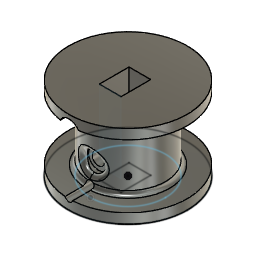
spool (Autodesk Fusion 360 design; units mm, degrees)
Autodesk Fusion 360 part; units mm, degrees
sketch "Skizze1" plane through (0, 0, 0) normal (0, 0, 1) x (1, 0, 0)
  circle A0 centre (0, 0) radius 15
  line L0 (-2.75, 3) -> (2.75, 3)
  line L1 (2.75, 3) -> (2.75, -4.5)
  line L2 (2.75, -4.5) -> (-2.75, -4.5)
  line L3 (-2.75, -4.5) -> (-2.75, 3)
  circle A1 centre (0, 0) radius 9.5
  point P0 (0, -9.5)
  dimension "d1" = 30
  dimension "d2" = 7.5
  dimension "d3" = 5.5
  dimension "d4" = 3
  dimension "d5" = 2.75
  dimension "d6" = 2.75
  dimension "d7" = 4.5
  dimension "d15" = 5
  constraint coincident A0.centre A1.centre
  constraint horizontal L0
  constraint vertical L1
  constraint horizontal L2
  constraint vertical L3
  constraint coincident A1 P0
  measures "d1" diameter of A0
  measures "d2" distance of L0 L2
  measures "d3" distance of L0.start L0.end
  measures "d4" distance of L0 A0.centre
  measures "d5" distance of L1 A0.centre
  measures "d6" distance of A0.centre L3
  measures "d7" distance of A0.centre L2
  measures "d15" distance of L2 P0
extrude "Extrusion1" add sketch "Skizze1" along normal blind 21 contours A0 | A1
extrude "Extrusion2" add sketch "Skizze1" along normal blind 3 contours L0 L1 L2 L3
hole "Bohrung1" at (0, 0, 0) direction (0, 0, 1) diameter 3.5 depth 6 tip angle 180
extrude "Extrusion3" cut sketch "Skizze1" along normal blind 16 from surface at 2.5 contours A0
sketch "Skizze2" plane through (0, -4.5, 0) normal (0, 1, 0) x (-1, 0, 0)
  line L0 (-2.75, 3) -> (2.75, 3)
  line L1 (2.75, 3) -> (2.75, 21)
  line L2 (2.75, 21) -> (-2.75, 21)
  line L3 (-2.75, 21) -> (-2.75, 3)
hole "Bohrung2" at (0, -9.5, 17.5) direction (0, 1, 0) diameter 3.1 depth 6 tip angle 180 counterbore diameter 5 counterbore depth 2
hole "Bohrung3" at (0, -9.5, 7.5) direction (0, 1, 0) diameter 3.1 depth 6 tip angle 180 counterbore diameter 5 counterbore depth 2
sketch "Skizze3" plane through (0, -4.5, 0) normal (0, 1, 0) x (-1, 0, 0)
  circle A0 centre (0, 17.5) radius 2.5
extrude "Extrusion4" cut sketch "Skizze3" against normal blind 11.5 from surface at -4.5
fillet "Abrundung1" radius 1 1 edges at (0, 9.5, 18.5) 1 faces at (-3.9607, -8.635, 7.8333)
sketch "Skizze4" plane through (0, 0, 0) normal (0, 1, 0) x (1, 0, 0)
  circle A0 centre (0, -2.8) radius 1
extrude "Extrusion5" cut sketch "Skizze4" against normal blind 20
